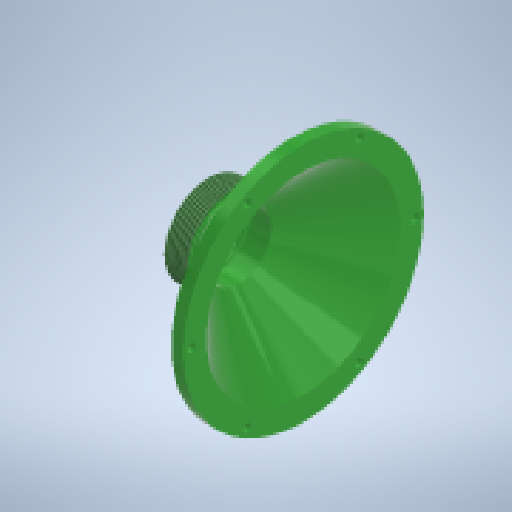
# Autodesk Inventor part: 027
Saved by Autodesk Inventor 2023 (Build 270158000, 158)
## iProperties
Created: 2022-04-04
Part Number: 027
Material: Aluminum 6061
Document SubType Name: Modeling
Designer: Vinicius Miguel
Density: 2.7 g/cm^3
Appearance: Smooth - Dark Forest Green
Mass: 41.2435 g
Surface Area: 84.7602 cm^2
Volume: 15.2754 cm^3
Author: Vinicius Miguel
Autodesk Inventor part; units mm, degrees
ref_plane "YZ Plane" through (0, 0, 0) normal (1, 0, 0) x (0, 1, 0)
ref_plane "XZ Plane" through (0, 0, 0) normal (0, 1, 0) x (-1, 0, 0)
ref_plane "XY Plane" through (0, 0, 0) normal (0, 0, 1) x (1, 0, 0)
sketch "Sketch1" plane through (0, 0, 0) normal (0, 1, 0) x (-1, 0, 0)
  line L0 (0, 0) -> (-9.3015, 0)
  line L1 (7.5, -14) -> (0, -14)
  line L2 (13, -19) -> (13, -16)
  line L3 (7.5, -16) -> (7.5, -14)
  line L4 (13, -19) -> (3, -19)
  line L5 (3, -19) -> (3, -17.4)
  line L6 (3, -17.4) -> (1, -17.4)
  line L7 (1, -17.4) -> (1, -19)
  line L8 (-22.5, -51.5) -> (-27.5, -51.5)
  line L9 (-27.5, -51.5) -> (-27.5, -41.5)
  line L10 (-27.5, -41.5) -> (0, -14)
  line L11 (13, -16) -> (11.5, -16)
  line L12 (11.5, -16) -> (11.5, -17)
  line L13 (11.5, -17) -> (10.5, -17)
  line L14 (10.5, -17) -> (10.5, -16)
  line L15 (10.5, -16) -> (7.5, -16)
  line L16 (-22.5, -51.5) -> (-22.5, -42.5)
  line L17 (-22.5, -42.5) -> (1, -19)
  point P0 (25, -13.6173)
  dimension "d2" = 28
  dimension "d19" = 103
  dimension "d20" = 83
  dimension "d21" = 5
  dimension "d22" = 1.6
  dimension "d23" = 135
  dimension "d24" = 2
  dimension "d25" = 1
  dimension "d26" = 1
  dimension "d27" = 3
  dimension "d28" = 1.5
  dimension "d29" = 38
  dimension "d30" = 2
  dimension "d32" = 10
  dimension "d33" = 9
  constraints: 36 end point, 10 perpendicular, 4 horizontal, 2 parallel, 2 point on line, 1 vertical, 1 vertical alignment
  measures "d2" diameter of L1 L0
  measures "d19" diameter of L8 L0
  measures "d20" diameter of L9.end L0
  measures "d21" distance of L8.start L8.end
  measures "d22" distance of L4.end L5.end
  measures "d23" angle of L10 L9
  measures "d24" distance of L5.end L6.end
  measures "d25" distance of L12.end L13.end
  measures "d26" distance of L11.end L12.end
  measures "d27" distance of L14.end L3.start
  measures "d28" distance of L2.end L11.end
  measures "d29" diameter of L4 L0
  measures "d30" distance between parallel lines of L4 L13
  measures "d32" distance of L2.start L4.end
  measures "d33" distance of L8.start L16.end
revolve "Revolution1" add sketch "Sketch1" angle 360 about axis through (0, 0, 0) along (1, 0, 0)
thread "Thread4" size "M38x1.5" class "6g" standard "ANSI Metric M Profile" full length
sketch "Sketch2" plane through (22.5, 0, 0) normal (-1, 0, 0) x (0, 0, 1)
  point P0 (0, 0)
  point P1 (48, 0)
  dimension "d36" = 48
  constraints: 1 horizontal alignment
  measures "d36" distance of point (0, 0) point (48, 0)
hole "Hole1" at (22.5, 0, 48) direction (1, 0, 0) diameter 3.5 depth 5
pattern_circular "Circular Pattern1" count 6 over 360 about axis through (25, 0, 0) along (1, 0, 0) of "Hole1"
body "Solid1"
